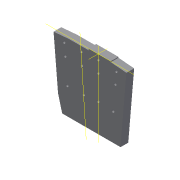
# Autodesk Inventor part: empty
Saved by Autodesk Inventor 2014 (Build 180170000, 170)
## iProperties
Created: 2015-04-13
Part Number: empty
Material: Generic
Document SubType Name: Modeling
Designer: Martin
Density: 1 g/cm^3
Appearance: Default
Author: Martin
Autodesk Inventor part; units mm, degrees
ref_plane "YZ Plane" through (0, 0, 0) normal (1, 0, 0) x (0, 1, 0)
ref_plane "XZ Plane" through (0, 0, 0) normal (0, 1, 0) x (-1, 0, 0)
sketch "Sketch1" plane through (0, 0, 0) normal (0, 1, 0) x (-1, 0, 0)
  line L0 (77, 0) -> (-56, 0) projected
  line L1 (0, -111.5403) -> (0, 39.2421) construction
  line L2 (58, 0) -> (-37, 0) construction
  line L3 (-37, 0) -> (-29.126, -90)
  line L4 (-29.126, -90) -> (46.5168, -90)
  line L5 (46.5168, -90) -> (51.8758, -70)
  line L6 (51.8758, -70) -> (58, 0)
  line L7 (0, -90) -> (0, -90) construction
  line L8 (-16.126, -90) -> (-24.0526, 0.6013) construction
  line L9 (37.126, -90) -> (46.4907, 17.039) construction
  circle A0 centre (44.2275, -8.8301) radius 1.75
  circle A1 centre (22.0675, -8.1849) radius 1.75
  circle A2 centre (0, -6.2) radius 1.75
  circle A3 centre (-23.315, -7.8301) radius 1.75
  circle A4 centre (42.9201, -23.773) radius 1.75
  circle A5 centre (21.0212, -23.1484) radius 1.75
  circle A6 centre (0, -21.2) radius 1.75
  circle A7 centre (-22.0076, -22.773) radius 1.75
  circle A8 centre (40.1486, -55.452) radius 1.75
  circle A9 centre (18.8029, -54.8709) radius 1.75
  circle A10 centre (0, -53) radius 1.75
  circle A11 centre (-19.2361, -54.452) radius 1.75
  line L10 (44.2275, -8.8301) -> (42.9201, -23.773)
  line L11 (22.0675, -8.1849) -> (21.0212, -23.1484)
  line L12 (0, -21.2) -> (0, -6.2)
  line L13 (-22.0076, -22.773) -> (-23.315, -7.8301)
  line L14 (42.9201, -23.773) -> (40.1486, -55.452)
  line L15 (0, -21.2) -> (0, -53)
  line L16 (-19.2361, -54.452) -> (-22.0076, -22.773)
  line L17 (21.0212, -23.1484) -> (18.8029, -54.8709)
  line L18 (12.3839, 0) -> (-16.3839, 0)
  line L19 (-16.3839, 0) -> (-16.3839, -1)
  line L20 (-16.3839, -1) -> (-36.7566, -2.7824)
  line L21 (12.3839, 0) -> (12.3839, -2)
  line L22 (12.3839, -2) -> (37.2964, -2)
  line L23 (37.2964, -2) -> (57.6691, -3.7824)
  line L24 (0, -6.2) -> (0, 0)
  line L25 (22.0675, -8.1849) -> (22.5, -2)
  line L26 (44.2275, -8.8301) -> (44.7678, -2.6537)
  line L27 (-23.315, -7.8301) -> (-23.8553, -1.6537)
  line L28 (16.3464, -90) -> (23.8777, 17.7017) construction
  point P0 (-24, 0)
  point P1 (25, 0)
  point P2 (45, 0)
  dimension "d0" = 95
  dimension "d1" = 37
  dimension "d2" = 24
  dimension "d3" = 25
  dimension "d4" = 45
  dimension "d5" = 5
  dimension "d7" = 5
  dimension "d8" = 105
  dimension "d9" = 20
  dimension "d10" = 90
  dimension "d11" = 3.5
  dimension "d12" = 31.8
  dimension "d13" = 15
  dimension "d14" = 2
  dimension "d15" = 1
  dimension "d16" = 7.5
  dimension "d18" = 7.5
  dimension "d19" = 6.2
  dimension "d22" = 4
  dimension "d23" = 22.5
  constraints: 54 end point, 32 point on line, 12 centre point, 11 equal radius, 9 collinear, 9 equal length, 5 perpendicular, 4 parallel
  measures "d0" distance of L2.end L2.start
  measures "d1" distance from line of L1 L2.end
  measures "d2" distance from line of L7 point (-24, 0)
  measures "d3" distance from line of L7 point (25, 0)
  measures "d4" distance from line of L7 point (45, 0)
  measures "d5" angle of L8 L7
  measures "d7" angle of L7 L9
  measures "d8" angle of L4 L5
  measures "d9" vertical distance of L4.end L5.end
  measures "d10" vertical distance of L3.end L2.end
  measures "d11" diameter of A3
  measures "d12" distance of L16.start L13.start
  measures "d13" distance of L13.start L13.end
  measures "d14" distance of L18.start L21.end
  measures "d15" distance of L18.end L19.end
  measures "d16" distance from line of L19.end L8
  measures "d18" distance from line of L22.end L9
  measures "d19" distance of L13.end L27.end
  measures "d22" angle of L1 L28
  measures "d23" distance from line of L1 L25.end
extrude "Extrusion1" add sketch "Sketch1" along normal blind 10 contours L21 L22 L23 L6 L5 L4 L3 L20 L19 L0
ref_plane "Work Plane1" through (-22.5, 0, -2) normal (-0.0697565, 0, 0.9975641) x (0, -1, 0)
body "Solid1"
